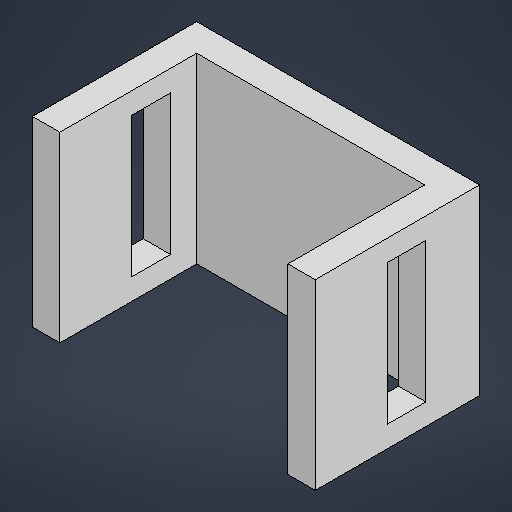
# Autodesk Inventor part: main
Saved by Autodesk Inventor 2026 (Build 300175050, 175E)
## iProperties
Created: 2025-09-02
Part Number: main
Material: 一般
Document SubType Name: Modeling
Designer: ka0n7
Density: 1 g/cm^3
Appearance: 既定
Author: ka0n7
Autodesk Inventor part; units mm, degrees
ref_plane "YZ Plane" through (0, 0, 0) normal (1, 0, 0) x (0, 1, 0)
ref_plane "XZ Plane" through (0, 0, 0) normal (0, 1, 0) x (-1, 0, 0)
ref_plane "XY Plane" through (0, 0, 0) normal (0, 0, 1) x (1, 0, 0)
sketch "スケッチ1" plane through (0, 0, 0) normal (0, 0, 1) x (1, 0, 0)
  line L0 (-31, 20) -> (31, 20)
  line L1 (31, 20) -> (31, -20)
  line L2 (31, -20) -> (-31, -20)
  line L3 (-31, -20) -> (-31, 20)
  line L4 (-31, 20) -> (31, -20) construction
  line L5 (31, 20) -> (-31, -20) construction
  point P0 (0, 0)
  dimension "d0" = 62
  dimension "d1" = 40
  constraints: 12 end point, 2 midpoint, 2 parallel, 1 horizontal, 1 perpendicular
  measures "d0" distance of L1.end L2.end
  measures "d1" distance of L0.end L1.end
extrude "押し出し1" add sketch "スケッチ1" along normal blind 6
sketch "スケッチ2" plane through (0, 0, 6) normal (0, 0, 1) x (1, 0, 0)
  line L0 (31, 20) -> (-31, 20) projected
  line L1 (-31, -20) -> (31, -20) projected
  line L2 (-31, 20) -> (-25, 20)
  line L3 (-25, 20) -> (-25, -20)
  line L4 (-25, -20) -> (-31, -20)
  line L5 (-31, -20) -> (-31, 20)
  line L6 (31, -20) -> (31, 20) projected
  line L7 (31, 20) -> (25, 20)
  line L8 (25, 20) -> (25, -20)
  line L9 (25, -20) -> (31, -20)
  line L10 (31, -20) -> (31, 20)
  point P0 (0, 0)
  dimension "d4" = 6
  dimension "d5" = 6
  constraints: 16 end point, 4 parallel, 2 horizontal, 2 perpendicular, 2 point on line
  measures "d4" distance between parallel lines of L5 L3
  measures "d5" distance between parallel lines of L6 L8
extrude "押し出し2" add sketch "スケッチ2" along normal blind 30 contours L6 L1 L8 L0 | L3 L1 L5 L0
sketch "スケッチ3" plane through (31, -20, 0) normal (1, 0, 0) x (0, 0, -1)
  line L0 (-6, 0) -> (-36, 0) projected
  line L1 (-18.303, 0) -> (-8.303, 0)
  line L2 (0, 0) -> (0, 40) projected
  line L3 (-36, 0) -> (-36, 40) projected
  line L4 (-36, 0) -> (-17.2102, 0)
  line L5 (0, 0) -> (-16, 0)
  line L6 (-16, 0) -> (-16, 20)
  line L7 (-16, 20) -> (0, 20)
  line L8 (0, 20) -> (0, 0)
  line L9 (-20.25, 35.337) -> (-11.75, 35.337)
  line L10 (-11.75, 35.337) -> (-11.75, 4.663)
  line L11 (-11.75, 4.663) -> (-20.25, 4.663)
  line L12 (-20.25, 4.663) -> (-20.25, 35.337)
  line L13 (-20.25, 35.337) -> (-11.75, 4.663) construction
  line L14 (-11.75, 35.337) -> (-20.25, 4.663) construction
  point P0 (0, 20)
  dimension "d9" = 36
  dimension "d10" = 40
  dimension "d11" = 20
  dimension "d12" = 16
  dimension "d13" = 8.5
  constraints: 24 end point, 4 parallel, 3 point on line, 2 horizontal, 2 midpoint, 2 perpendicular
  measures "d9" distance between parallel lines of L2 L3
  measures "d10" distance of L0.end L3.end
  measures "d11" distance of L5.end L6.end
  measures "d12" distance of L6.end L7.end
  measures "d13" distance of L10.end L11.end
extrude "押し出し3" cut sketch "スケッチ3" against normal blind 100 contours L11 L12 L9 L10 L7 L6 | L6 L7 L10 L11
equation "\"d5\" = d4"
equation "\"d11\" = 0.5 * d10"
